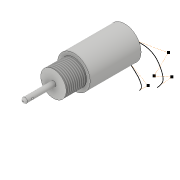
# Autodesk Inventor part: dc motor
Saved by Autodesk Inventor 2019 (Build 230136000, 136)
## iProperties
Created: 2019-10-07
Part Number: dc motor
Material: Generic
Document SubType Name: Modeling
Designer: Admin
Density: 1 g/cm^3
Appearance: Default
Author: Admin
Autodesk Inventor part; units mm, degrees
ref_plane "YZ Plane" through (0, 0, 0) normal (1, 0, 0) x (0, 1, 0)
ref_plane "XZ Plane" through (0, 0, 0) normal (0, 1, 0) x (-1, 0, 0)
ref_plane "XY Plane" through (0, 0, 0) normal (0, 0, 1) x (1, 0, 0)
sketch "Sketch1" plane through (0, 0, 0) normal (0, 0, 1) x (1, 0, 0)
  circle A0 centre (0, 0) radius 16
  dimension "d0" = 32
  constraints: 1 centre point, 1 coincident
  measures "d0" diameter of A0
extrude "Extrusion1" add sketch "Sketch1" along normal blind 50
sketch "Sketch2" plane through (0, 0, 50) normal (0, 0, 1) x (1, 0, 0)
  circle A0 centre (0, 0) radius 12.5
  dimension "d3" = 25
  constraints: 1 centre point, 1 coincident
  measures "d3" diameter of A0
extrude "Extrusion2" add sketch "Sketch2" along normal blind 20
thread "Thread1" size "M25x2" class "6g" standard "ANSI Metric M Profile" full length
sketch "Sketch3" plane through (0, 0, 70) normal (0, 0, 1) x (1, 0, 0)
  circle A0 centre (0, 0) radius 2.5
  dimension "d8" = 5
  constraints: 1 centre point, 1 coincident
  measures "d8" diameter of A0
extrude "Extrusion3" add sketch "Sketch3" along normal blind 30
sketch "Sketch4" plane through (0, 0, 0) normal (1, 0, 0) x (0, 1, 0)
  line L0 (2.5, 100) -> (-2.5, 100) projected
  line L1 (0, 100) -> (0, 93)
  circle A0 centre (0, 93) radius 1
  point P0 (0, 0)
  dimension "d11" = 7
  dimension "d12" = 2
  constraints: 2 end point, 1 centre point, 1 coincident, 1 midpoint, 1 vertical
  measures "d11" distance of L1.start L1.end
  measures "d12" diameter of A0
extrude "Extrusion4" cut sketch "Sketch4" along normal through all both and the other way through all
fillet "Fillet1" radius 2 1 edges at (-2.5, 0, 100)
sketch "Sketch5" plane through (0, 0, 0) normal (0, 0, 1) x (1, 0, 0)
  circle A0 centre (6.35, 6.35) radius 0.5
  circle A1 centre (-7.9375, -6.35) radius 0.5
  point P0 (0, 0)
  dimension "d16" = 1
  dimension "d17" = 1
  constraints: 2 centre point
  measures "d16" diameter of A0
  measures "d17" diameter of A1
extrude "Extrusion5" add sketch "Sketch5" against normal blind 1.7 contours A0
sketch "Sketch6" plane through (0, 0, 0) normal (0, 0, -1) x (-1, 0, 0)
  circle A0 centre (6.35, -7.9375) radius 0.5
  point P0 (0, 0)
  dimension "d20" = 1
  constraints: 1 centre point
  measures "d20" diameter of A0
extrude "Extrusion6" add sketch "Sketch6" along normal blind 1.7
sketch "Sketch7" plane through (0, 0, 0) normal (0, 0, -1) x (-1, 0, 0)
  circle A0 centre (-6.35, 6.35) radius 0.5 projected
  line L0 (-6.35, 6.35) -> (-42.8625, 12.7) construction
  line L1 (-42.8625, 12.7) -> (-28.575, -14.2875) construction
  line L2 (-28.575, -14.2875) -> (-46.0375, -6.35) construction
  line L3 (-46.0375, -6.35) -> (-31.75, -22.225) construction
  spline S0 degree 4 poles (-6.35, 6.35) (-42.8625, 12.7) (-28.575, -14.2875) (-46.0375, -6.35) (-31.75, -22.225) knots 1 1 1 1 1 2 2 2 2 2
  line L4 (6.35, -7.9375) -> (-22.6919, -25.4) construction
  line L5 (-22.6919, -25.4) -> (-14.2875, -33.3375) construction
  spline S1 degree 2 poles (6.35, -7.9375) (-22.6919, -25.4) (-14.2875, -33.3375) knots 1 1 1 2 2 2
  point P0 (0, 0)
  constraints: 6 other
body "Solid1"
